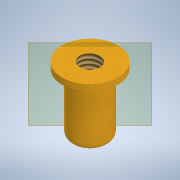
# Autodesk Inventor part: M4 Rivet nut
Saved by Autodesk Inventor 2020.3 (Build 243373000, 373)
## iProperties
Created: 2020-06-30
Part Number: M4 Rivet nut
Material: Brass, Soft Yellow, Welded
Document SubType Name: Modeling
Designer: Bruno
Density: 8.5 g/cm^3
Appearance: Weld - Brass
Author: Bruno
Autodesk Inventor part; units mm, degrees
ref_plane "YZ Plane" through (0, 0, 0) normal (1, 0, 0) x (0, 1, 0)
ref_plane "XZ Plane" through (0, 0, 0) normal (0, 1, 0) x (-1, 0, 0)
ref_plane "XY Plane" through (0, 0, 0) normal (0, 0, 1) x (1, 0, 0)
sketch "Sketch1" plane through (0, 0, 0) normal (0, 0, 1) x (1, 0, 0)
  line L0 (0, 0) -> (2.95, 0)
  line L1 (2.95, 0) -> (2.95, 9.5)
  line L2 (0, 0) -> (0, 10.5)
  line L3 (0, 10.5) -> (4.5, 10.5)
  line L4 (4.5, 10.5) -> (4.5, 9.5)
  line L5 (4.5, 9.5) -> (2.95, 9.5)
  dimension "d0" = 2.95
  dimension "d1" = 9.5
  dimension "d2" = 10.5
  dimension "d3" = 4.5
  constraints: 12 end point, 4 perpendicular, 1 horizontal, 1 vertical
  measures "d0" distance of L0.start L0.end
  measures "d1" distance of L0.end L1.end
  measures "d2" distance of L0.start L2.end
  measures "d3" distance of L2.end L3.end
revolve "Revolution1" add sketch "Sketch1" angle 360 about axis through (0, 0, 0) along (0, 1, 0)
sketch "Sketch2" plane through (0, 10.5, 0) normal (0, 1, 0) x (1, 0, 0)
  point P0 (0, 0)
  point P1 (0, 0)
  constraints: 1 coincident, 1 other
hole "Hole1" at (0, 10.5, 0) direction (0, -1, 0) diameter 3.242 end through all thread size "M4x0.7" class "6H" standard "ISO Metric profile"
fillet "Fillet1" radius 1 1 edges at (-2.95, 0, 0)
body "Solid1"
